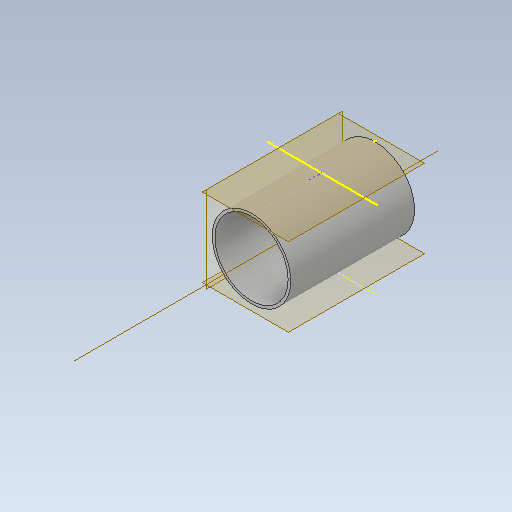
# Autodesk Inventor part: CF9512_mounting_lugs
Saved by Autodesk Inventor 2020.5 (Build 245400000, 400)
## iProperties
Created: 2018-05-08
Part Number: CF9512_mounting_lugs
Material: Generic
Document SubType Name: Modeling
Designer: rainer
Density: 1 g/cm^3
Appearance: Default
Author: rainer
Autodesk Inventor part; units mm, degrees
ref_plane "XY Plane" through (0, 0, 0) normal (0, 0, 1) x (1, 0, 0)
sketch "Sketch1" plane through (0, 0, 0) normal (0, 0, 1) x (1, 0, 0)
  circle A0 centre (0, 0) radius 128.6
  dimension "d0" = 257.2
  constraints: 1 centre point, 1 coincident
  measures "d0" diameter of A0
extrude "Extrusion1" add sketch "Sketch1" along normal blind 406
sketch "Sketch2" plane through (0, 0, 406) normal (0, 0, 1) x (1, 0, 0)
  circle A0 centre (0, 0) radius 120
  dimension "d3" = 240
  constraints: 1 centre point, 1 coincident
  measures "d3" diameter of A0
extrude "Extrusion2" cut sketch "Sketch2" against normal blind 305
ref_plane "Work Plane1" through (0, 0, 176) normal (0, 0, 1) x (1, 0, 0)
ref_plane "Work Plane2" through (0, 125, 0) normal (0, 1, 0) x (-1, 0, 0)
ref_plane "Work Plane3" through (0, -125, 0) normal (0, 1, 0) x (-1, 0, 0)
ref_plane "Work Plane4" through (-125, 0, 0) normal (1, 0, 0) x (0, 1, 0)
ref_plane "Work Plane5" through (0, 128.6, 0) normal (0, 1, 0) x (-1, 0, 0)
sketch "Sketch5" plane through (0, 128.6, 0) normal (0, 1, 0) x (-1, 0, 0)
  line L0 (-180.04, 176) -> (180.04, 176) projected
  line L1 (0, 176) -> (0, 218.6264) construction
  point P0 (0, 0)
  constraints: 2 end point, 1 midpoint, 1 perpendicular
ref_plane "Work Plane6" through (-128.6, 0, 0) normal (1, 0, 0) x (0, 1, 0)
sketch "Sketch6" plane through (-128.6, 0, 0) normal (1, 0, 0) x (0, 1, 0)
  line L0 (0, 175.878) -> (0, 199.156) construction
  point P0 (0, 0)
  constraints: 2 end point, 1 vertical
ref_plane "Work Plane7" through (0, -128.6, 0) normal (0, 1, 0) x (-1, 0, 0)
sketch "Sketch7" plane through (0, -128.6, 0) normal (0, 1, 0) x (-1, 0, 0)
  line L0 (-180.04, 176) -> (180.04, 176) construction
  line L1 (0, 176) -> (0, 205.0219) construction
  point P0 (0, 0)
  constraints: 2 end point, 1 midpoint, 1 vertical
sketch "Sketch8" plane through (0, 0, 101) normal (0, 0, 1) x (1, 0, 0)
  point P0 (0, 0)
  point P1 (0, 0)
  constraints: 1 coincident
body "Solid1"
